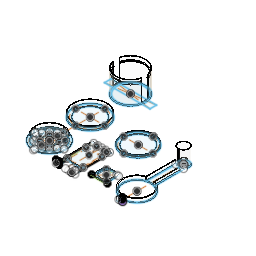
CAPV5 v1 (Autodesk Fusion 360 design; units mm, degrees)
Autodesk Fusion 360 part; units mm, degrees
sketch "Sketch1" plane through (0, 0, 0) normal (0, 0, 1) x (1, 0, 0) in component "Component"
  circle A0 centre (50, 50) radius 41.5
  circle A1 centre (50, 50) radius 18.25
  line L0 (65, 65) -> (35, 65) construction
  line L1 (35, 65) -> (35, 35) construction
  line L2 (35, 35) -> (65, 35) construction
  line L3 (65, 35) -> (65, 65) construction
  line L4 (65, 65) -> (35, 35) construction
  line L5 (35, 65) -> (65, 35) construction
  circle A2 centre (65, 35) radius 1.75
  circle A3 centre (65, 65) radius 1.75
  circle A4 centre (35, 65) radius 1.75
  circle A5 centre (35, 35) radius 1.75
  circle A6 centre (50, 25.5) radius 1.6
  circle A7 centre (50, 74.5) radius 1.6
  line L6 (69.5, 30.5) -> (30.5, 30.5) construction
  line L7 (30.5, 30.5) -> (30.5, 69.5) construction
  line L8 (30.5, 69.5) -> (69.5, 69.5) construction
  line L9 (69.5, 69.5) -> (69.5, 30.5) construction
  line L10 (69.5, 30.5) -> (30.5, 69.5) construction
  line L11 (30.5, 30.5) -> (69.5, 69.5) construction
  line L12 (120, 0) -> (130, 0)
  line L13 (120, 111.4151) -> (120, 0)
  line L14 (169, 0) -> (179, 0)
  line L15 (179, 0) -> (179, 111.4151)
  line L16 (120, 30) -> (179, 30) construction
  line L17 (120, 88) -> (179, 88) construction
  line L18 (125, 0) -> (125, 111.5) construction
  line L19 (174, 0) -> (174, 111.5) construction
  circle A8 centre (125, 30) radius 1.75
  circle A9 centre (174, 30) radius 1.75
  circle A10 centre (125, 88) radius 1.75
  circle A11 centre (174, 88) radius 1.75
  line L20 (50, 50) -> (50, 0) construction
  line L21 (50, 50) -> (50, 93.5) construction
  line L22 (130, 25.5) -> (169, 25.5)
  line L23 (149.5, 111.5) -> (149.5, 0) construction
  line L24 (50, 93.5) -> (50, 225.5598) construction
  circle A12 centre (50, 175.4598) radius 50.1
  circle A13 centre (50, 175.4598) radius 52.1
  circle A14 centre (50, 175.4598) radius 40.1
  circle A15 centre (58.774, 82.7449) radius 5
  circle A16 centre (41.226, 82.7449) radius 5
  circle A17 centre (26.0291, 73.9709) radius 5
  circle A18 centre (17.2551, 58.774) radius 5
  circle A19 centre (17.2551, 41.226) radius 5
  circle A20 centre (26.0291, 26.0291) radius 5
  circle A21 centre (41.226, 17.2551) radius 5
  circle A22 centre (58.774, 17.2551) radius 5
  circle A23 centre (73.9709, 26.0291) radius 5
  circle A24 centre (82.7449, 41.226) radius 5
  circle A25 centre (82.7449, 58.774) radius 5
  circle A26 centre (73.9709, 73.9709) radius 5
  circle A27 centre (65, 35) radius 3
  circle A28 centre (65, 65) radius 3
  circle A29 centre (35, 35) radius 3
  circle A30 centre (35, 65) radius 3
  line L25 (120, 10) -> (130, 10)
  line L26 (169, 10) -> (179, 10)
  line L27 (130, 0) -> (130, 25.5)
  line L28 (169, 25.5) -> (169, 0)
  line L29 (138, 107.4151) -> (138, 111.5) construction
  line L30 (161.05, 107.4151) -> (161.05, 111.5) construction
  line L31 (120, 107.4151) -> (179, 107.4151) construction
  line L32 (120, 111.4151) -> (179, 111.4151)
  circle A31 centre (138, 107.4151) radius 1.7
  circle A32 centre (149.5, 72.4151) radius 1.7
  line L33 (120, 90.4151) -> (179, 90.4151) construction
  circle A33 centre (135.5, 90.4151) radius 1.7
  line L34 (171, 88) -> (171, 30) construction
  line L35 (177, 30) -> (177, 88) construction
  line L36 (122, 30) -> (122, 88) construction
  line L37 (128, 30) -> (128, 88) construction
  line L38 (128, 75.2678) -> (128, 75.2679) construction
  line L39 (128, 75.2678) -> (128, 75.2679)
  circle A34 centre (161.05, 107.4151) radius 1.7
  circle A35 centre (50, 50) radius 50
  circle A36 centre (50, 175.4598) radius 45 construction
  line L40 (50, 175.4598) -> (102.1, 175.4598) construction
  line L41 (50, 175.4598) -> (-2.1, 175.4598) construction
  circle A37 centre (50, 220.4598) radius 1.6
  circle A38 centre (95, 175.4598) radius 1.6
  circle A39 centre (50, 130.4598) radius 1.6
  circle A40 centre (5, 175.4598) radius 1.6
  circle A41 centre (50, 50) radius 45 construction
  circle A42 centre (50, 95) radius 2.05
  circle A43 centre (4.9633, 50.0341) radius 2.05
  circle A44 centre (49.9642, 4.9627) radius 2.05
  circle A45 centre (95.0328, 50.0188) radius 2.05
  arc A46 (48.6263, 93.4783) -> (6.5215, 51.3662) centre (50, 50) ccw
  arc A47 (6.5193, 48.6993) -> (48.6327, 6.5214) centre (50, 50) ccw
  arc A48 (51.2973, 6.52) -> (93.4763, 48.6847) centre (50.0149, 49.9818) ccw
  arc A49 (93.4741, 51.3504) -> (51.333, 93.4426) centre (50.0149, 49.9818) ccw
  circle A50 centre (50, 50) radius 33.9 construction
  circle A51 centre (50, 50) radius 38.9 construction
  circle A52 centre (198.4118, 175.4598) radius 45 construction
  line L42 (198.4118, 175.4598) -> (247.9118, 175.4598) construction
  circle A53 centre (198.4118, 175.4598) radius 40.1
  circle A54 centre (243.4118, 175.4598) radius 1.6
  circle A55 centre (198.4118, 130.4598) radius 1.6
  circle A56 centre (198.4118, 220.4598) radius 1.6
  circle A57 centre (153.4118, 175.4598) radius 1.6
  circle A58 centre (198.4118, 175.4598) radius 49.5
  line L43 (198.4118, 175.4598) -> (148.9118, 175.4598) construction
  circle A59 centre (198.4118, 175.4598) radius 47.6
  circle A60 centre (168.5, 107.4151) radius 1.7
  line L44 (320, 50) -> (320, -0.2775) construction
  line L45 (321.5, 8.5271) -> (321.5, -6.2719)
  line L46 (318.5, 8.5271) -> (318.5, -6.2719)
  arc A61 (321.5, 8.5271) -> (318.5, 8.5271) centre (320, 50) ccw
  line L47 (314.5, 5.8412) -> (314.5, -6.2719)
  line L48 (325.5, 5.8412) -> (325.5, -6.2719)
  line L49 (314.5, -6.2719) -> (318.5, -6.2719)
  line L50 (321.5, -6.2719) -> (325.5, -6.2719)
  line L51 (314, -0.2719) -> (327, -0.2719) construction
  line L52 (320, 50) -> (320, 193.7281) construction
  line L53 (317, 193.7281) -> (323, 193.7281)
  circle A62 centre (320.0004, 193.6763) radius 7.45
  line L54 (332, 89.7272) -> (332, 181.6865)
  line L55 (308, 89.7272) -> (308, 181.6865)
  arc A63 (322, 178.862) -> (318, 178.862) centre (320, 193.7281) ccw
  arc A64 (322, 176.8462) -> (318, 176.8462) centre (320, 193.7281) ccw
  line L56 (334, 92.2404) -> (334, 184.0845)
  line L57 (306, 92.2404) -> (306, 184.0845)
  arc A65 (325.5, 5.8412) -> (334, 92.2404) centre (320, 50) ccw
  arc A66 (306, 92.2404) -> (314.5, 5.8412) centre (320, 50) ccw
  arc A67 (332, 92.8515) -> (308, 92.8515) centre (320, 50) ccw
  circle A68 centre (320, 193.7281) radius 9.5
  line L58 (318, 176.8462) -> (322, 176.8462)
  line L59 (318, 178.862) -> (322, 178.862)
  line L60 (322, 176.8462) -> (322, 178.862)
  line L61 (322, 184.441) -> (322, 186.4997)
  line L62 (318, 176.8462) -> (318, 178.862)
  line L63 (318, 184.441) -> (318, 186.4999)
  line L64 (251, 28.5) -> (257.5, 28.5)
  line L65 (229.5, 65) -> (229.5, 21.5) construction
  line L66 (245.5, 62) -> (245.5, 30) construction
  circle A69 centre (245.5, 30) radius 2.75
  line L67 (213.5, 62) -> (213.5, 30) construction
  circle A70 centre (213.5, 62) radius 2.75
  line L68 (208, 28.5) -> (208, 66.5)
  line L69 (213.5, 30) -> (245.5, 62) construction
  line L70 (208, 62) -> (251, 62) construction
  line L71 (245.5, 30) -> (213.5, 62) construction
  line L72 (251, 28.5) -> (251, 66.5)
  circle A71 centre (125, 30) radius 3
  circle A72 centre (174, 30) radius 3
  circle A73 centre (125, 88) radius 3
  circle A74 centre (174, 88) radius 3
  line L73 (208, 30) -> (251, 30) construction
  line L74 (208, 66.5) -> (251, 66.5)
  circle A75 centre (229.5, 46) radius 19
  circle A76 centre (50, 300) radius 44.25
  circle A77 centre (50, 300) radius 46.25
  circle A78 centre (50, 300) radius 41.25
  line L75 (120, 290) -> (-20, 290)
  line L76 (-20, 290) -> (-20, 310)
  line L77 (-20, 310) -> (120, 310)
  line L78 (120, 310) -> (120, 290)
  line L79 (120, 290) -> (-20, 310) construction
  line L80 (-20, 290) -> (120, 310) construction
  line L81 (201.5, 25) -> (257.5, 25) construction
  circle A79 centre (205, 25) radius 1.4
  circle A80 centre (254, 25) radius 1.4
  line L82 (201.5, 21.5) -> (257.5, 21.5)
  line L83 (257.5, 28.5) -> (257.5, 21.5)
  line L84 (251, 28.5) -> (201.5, 28.5) construction
  line L85 (208, 28.5) -> (201.5, 28.5)
  line L86 (201.5, 28.5) -> (201.5, 21.5)
  arc A81 (53.6265, 93.3123) -> (46.3574, 93.3472) centre (50, 95) ccw
  arc A82 (6.6542, 53.6591) -> (6.6486, 46.4064) centre (4.9633, 50.0341) ccw
  arc A83 (46.3394, 6.6542) -> (53.5916, 6.6484) centre (49.9642, 4.9627) ccw
  arc A84 (93.3472, 46.3913) -> (93.3412, 53.6436) centre (95.0328, 50.0188) ccw
  point P0 (50, 50)
  point P1 (50, 50)
  point P2 (50, 25.5)
  point P3 (50, 74.5)
  point P4 (50, 25.5)
  point P5 (50, 74.5)
  point P6 (50, 50)
  point P7 (120, 0)
  point P8 (169, 0)
  point P9 (149.5, 72.4151)
  point P10 (50, 50)
  point P11 (198.4118, 223.0598)
  point P12 (168.5, 107.4151)
  point P13 (320, 50)
  point P14 (320, 50)
  point P15 (50, 300)
  dimension "d3" = 83
  dimension "d4" = 36.5
  dimension "d12" = 30
  dimension "d13" = 30
  dimension "d14" = 3.5
  dimension "d15" = 3.5
  dimension "d16" = 3.5
  dimension "d17" = 3.5
  dimension "d18" = 24.5
  dimension "d19" = 24.5
  dimension "d28" = 3.2
  dimension "d29" = 3.2
  dimension "d30" = 39
  dimension "d31" = 39
  dimension "d61" = 10
  dimension "d63" = 10
  dimension "d66" = 30
  dimension "d67" = 58
  dimension "d68" = 3.5
  dimension "d69" = 3.5
  dimension "d70" = 3.5
  dimension "d71" = 3.5
  dimension "d80" = 49
  dimension "d93" = 4.5
  dimension "d109" = 87
  dimension "d110" = 100.2
  dimension "d111" = 104.2
  dimension "d112" = 80.2
  dimension "d120" = 77.8
  dimension "d123" = 6
  dimension "d124" = 6
  dimension "d125" = 6
  dimension "d126" = 6
  dimension "d150" = 4
  dimension "d151" = 3.4
  dimension "d153" = 35
  dimension "d154" = 3.4
  dimension "d166" = 3.4
  dimension "d190" = 3.4
  dimension "d199" = 100
  dimension "d200" = 90
  dimension "d201" = 3.2
  dimension "d202" = 3.2
  dimension "d203" = 3.2
  dimension "d204" = 3.2
  dimension "d205" = 90
  dimension "d206" = 4.1
  dimension "d222" = 95.2
  dimension "d223" = 99
  dimension "d224" = 80.2
  dimension "d225" = 90
  dimension "d226" = 3.2
  dimension "d227" = 3.2
  dimension "d228" = 3.2
  dimension "d229" = 3.2
  dimension "d243" = 33
  dimension "d244" = 3.4
  dimension "d248" = 10.5
  dimension "d249" = 17
  dimension "d250" = 83
  dimension "d251" = 89
  dimension "d254" = 4
  dimension "d255" = 4
  dimension "d260" = 200
  dimension "d261" = 30
  dimension "d265" = 14.9
  dimension "d266" = 19
  dimension "d267" = 2
  dimension "d268" = 2
  dimension "d270" = 34
  dimension "d316" = 10
  dimension "d353" = 16
  dimension "d354" = 5.5
  dimension "d357" = 5.5
  dimension "d358" = 38
  dimension "d371" = 6
  dimension "d372" = 6
  dimension "d373" = 6
  dimension "d374" = 6
  dimension "d389" = 88.5
  dimension "d390" = 92.5
  dimension "d391" = 82.5
  dimension "d409" = 20
  dimension "d416" = 2.8
  dimension "d418" = 2.8
  dimension "d421" = 3.5
  dimension "d423" = 3.5
  dimension "d424" = 3.5
  dimension "d425" = 3.5
  dimension "d432" = 24.5
  dimension "d433" = 24.5
  dimension "d434" = 45
  dimension "d435" = 4.1
  dimension "d436" = 4.1
  dimension "d437" = 4.1
  dimension "d442" = 8
  dimension "d443" = 8
  dimension "d444" = 8
  dimension "d445" = 8
  constraint coincident P10 P6
  constraint concentric A0 A1
  constraint horizontal L0
  constraint perpendicular L0 L1
  constraint parallel L0 L2
  constraint parallel L1 L3
  constraint coincident L4 P10
  constraint coincident L5 P10
  constraint coincident L2.end L3.start
  constraint coincident L0.start L3.end
  constraint coincident L0.end L1.start
  constraint coincident L1.end L2.start
  constraint coincident P4 P2
  constraint coincident P5 P3
  constraint horizontal L6
  constraint perpendicular L6 L7
  constraint parallel L6 L8
  constraint parallel L7 L9
  constraint coincident L10 P10
  constraint coincident L11 P10
  constraint horizontal P7 P8
  constraint horizontal L12
  constraint vertical L27
  constraint vertical L13
  constraint coincident P7 L12.start
  constraint horizontal L14
  constraint vertical L15
  constraint coincident P8 L14.start
  constraint coincident L13 L16.start
  constraint coincident L15 L16.end
  constraint perpendicular L15 L16
  constraint coincident L13 L17.start
  constraint coincident L15 L17.end
  constraint perpendicular L15 L17
  constraint midpoint L12 L18.start
  constraint midpoint L14 L19.start
  constraint coincident L18 A8.centre
  constraint coincident L16 A8.centre
  constraint coincident L19 A9.centre
  constraint coincident L16 A9.centre
  constraint coincident L17 A10.centre
  constraint coincident L18 A10.centre
  constraint coincident L17 A11.centre
  constraint coincident L19 A11.centre
  constraint perpendicular L2 L20
  constraint vertical L21
  constraint perpendicular L16 L23
  constraint parallel L21 L24
  constraint coincident L24 A12.centre
  constraint concentric A12 A13
  constraint concentric A13 A14
  constraint concentric A1 A51
  constraint concentric A2 A27
  constraint concentric A3 A28
  constraint concentric A5 A29
  constraint concentric A4 A30
  constraint coincident L13 L25.start
  constraint coincident L15 L26.end
  constraint perpendicular L15 L25
  constraint coincident L25.end L27
  constraint collinear L25 L26
  constraint coincident L13 L31.start
  constraint coincident L15 L31.end
  constraint perpendicular L15 L31
  constraint perpendicular L15 L32
  constraint coincident L31 L29.start
  constraint coincident L23 P9
  constraint coincident P9 A32.centre
  constraint coincident L13 L33.start
  constraint coincident L15 L33.end
  constraint perpendicular L15 L33
  constraint coincident L17 L34.start
  constraint coincident L16 L34.end
  constraint coincident L16 L35.start
  constraint coincident L17 L35.end
  constraint coincident L16 L36.start
  constraint coincident L17 L36.end
  constraint coincident L16 L37.start
  constraint coincident L37 L38.start
  constraint coincident L37 L38.end
  constraint coincident L31 L30.start
  constraint concentric A12 A36
  constraint coincident A12 L24.end
  constraint coincident A12.centre A13.centre
  constraint coincident A13 L40.end
  constraint horizontal L40
  constraint coincident A13 L41.end
  constraint horizontal L41
  constraint coincident A36 A37.centre
  constraint coincident L24 A37.centre
  constraint coincident A36 A38.centre
  constraint coincident L40 A38.centre
  constraint coincident A36 A39.centre
  constraint coincident L24 A39.centre
  constraint coincident A36 A40.centre
  constraint coincident L41 A40.centre
  constraint concentric A0 A41
  constraint coincident A41 A42.centre
  constraint coincident L24 A42.centre
  constraint concentric A46 A47
  constraint concentric A48 A49
  constraint coincident A45 A48.end
  constraint coincident A45 A49.start
  constraint coincident A44 A48.start
  constraint coincident A44 A47.end
  constraint coincident A43 A47.start
  constraint coincident A43 A46.end
  constraint coincident A42 A49.end
  constraint coincident A42 A46.start
  constraint coincident A26.centre A50
  constraint concentric A58 A59
  constraint concentric A53 A58
  constraint concentric A52 A59
  constraint coincident P11 A59
  constraint coincident A52.centre L42.start
  constraint coincident L42.end A58
  constraint horizontal L42
  constraint coincident L43.end A58
  constraint horizontal L43
  constraint coincident A56.centre A52
  constraint coincident A54.centre A52
  constraint coincident A54.centre L42
  constraint coincident A55.centre A52
  constraint coincident A57.centre A52
  constraint coincident A57.centre L43
  constraint coincident L31 P12
  constraint coincident P12 A60.centre
  constraint concentric A61 A65
  constraint coincident P14 P13
  constraint vertical L44
  constraint vertical L45
  constraint vertical L46
  constraint perpendicular L48 L49
  constraint coincident L45.end L49
  constraint collinear L49 L50
  constraint perpendicular L44 L51
  constraint parallel L44 L52
  constraint coincident L52.end A63.centre
  constraint perpendicular L53 L60
  constraint coincident A67.end A65
  constraint coincident A67.start A65
  constraint concentric A63 A64
  constraint coincident A64 L56.end
  constraint coincident A64 L57.end
  constraint coincident L57.start A65
  constraint concentric A65 A67
  constraint concentric A66 A67
  constraint coincident A62 L61.end
  constraint coincident A62 L63.end
  constraint coincident A68 L61.start
  constraint collinear L60 L61
  constraint coincident A68 L63.start
  constraint collinear L62 L63
  constraint coincident A61 L55.start
  constraint coincident L55 A67.end
  constraint coincident A61 L54.start
  constraint coincident L54 A67.start
  constraint coincident L67.start L70
  constraint coincident L66.start L70
  constraint perpendicular L66 L70
  constraint coincident L67.start A70.centre
  constraint coincident L66.end A69.centre
  constraint perpendicular L69 L71
  constraint midpoint A75.centre L69
  constraint concentric A8 A71
  constraint concentric A9 A72
  constraint concentric A10 A73
  constraint concentric A11 A74
  constraint coincident L68 L70.start
  constraint coincident L68 L73.start
  constraint concentric A76 A77
  constraint concentric A76 A78
  constraint horizontal L75
  constraint perpendicular L75 L76
  constraint parallel L75 L77
  constraint parallel L76 L78
  constraint coincident L79 P15
  constraint coincident L80 P15
  constraint coincident P15 A76.centre
  constraint perpendicular L67 L81
  constraint coincident L81 A79.centre
  constraint coincident L81 A80.centre
  constraint horizontal L82
  constraint perpendicular L82 L83
  constraint coincident L83 L81.end
  constraint perpendicular L68 L84
  constraint coincident L84 L68.start
  constraint perpendicular L82 L86
  constraint coincident L86 L81.start
  constraint coincident L82 L65.end
  constraint coincident L72 L73.end
  constraint coincident A75 L65.start
  constraint coincident A46 A81.end
  constraint coincident A49 A81.start
  constraint concentric A43 A82
  constraint coincident A46 A82.start
  constraint coincident A47 A82.end
  constraint concentric A44 A83
  constraint coincident A47 A83.start
  constraint coincident A48 A83.end
  constraint concentric A45 A84
  constraint coincident A49 A84.end
  constraint coincident A48 A84.start
  measures "d3" diameter of A0
  measures "d4" diameter of A1
  measures "d12" distance of L1.end L2.end
  measures "d13" distance of L0.end L1.end
  measures "d14" diameter of A2
  measures "d15" diameter of A3
  measures "d16" diameter of A4
  measures "d17" diameter of A5
  measures "d18" distance of P10 P4
  measures "d19" distance of P10 P5
  measures "d28" diameter of A6
  measures "d29" diameter of A7
  measures "d30" distance of L7.end L8.end
  measures "d31" distance of L6.end L7.end
  measures "d61" distance of P7 L12.end
  measures "d63" distance of P8 L14.end
  measures "d66" distance of L14.end L16.end
  measures "d67" distance of L16.end L17.end
  measures "d68" diameter of A8
  measures "d69" diameter of A9
  measures "d70" diameter of A10
  measures "d71" diameter of A11
  measures "d80" distance of L18.start L19.start
  measures "d93" distance of L16 L22
  measures "d109" diameter of A46
  measures "d110" diameter of A12
  measures "d111" diameter of A13
  measures "d112" diameter of A14
  measures "d120" diameter of A51
  measures "d123" diameter of A27
  measures "d124" diameter of A28
  measures "d125" diameter of A29
  measures "d126" diameter of A30
  measures "d150" distance of L15.end L31.end
  measures "d151" diameter of A31
  measures "d153" distance of L31 P9
  measures "d154" diameter of A32
  measures "d166" diameter of A33
  measures "d190" diameter of A34
  measures "d199" diameter of A35
  measures "d200" diameter of A36
  measures "d201" diameter of A37
  measures "d202" diameter of A38
  measures "d203" diameter of A39
  measures "d204" diameter of A40
  measures "d205" diameter of A41
  measures "d206" diameter of A42
  measures "d222" diameter of A59
  measures "d223" diameter of A58
  measures "d224" diameter of A53
  measures "d225" diameter of A52
  measures "d226" diameter of A56
  measures "d227" diameter of A54
  measures "d228" diameter of A55
  measures "d229" diameter of A57
  measures "d243" horizontal distance of A33.centre P12
  measures "d244" diameter of A60
  measures "d248" distance of L18 A33.centre
  measures "d249" distance of L31 L33
  measures "d250" diameter of A61
  measures "d251" diameter of A65
  measures "d254" distance of L46 L47
  measures "d255" distance of L45 L48
  measures "d260" vertical distance of L48.end L52.end
  measures "d261" diameter of A63
  measures "d265" diameter of A62
  measures "d266" diameter of A68
  measures "d267" distance of L52 L60
  measures "d268" distance of L52 L62
  measures "d270" diameter of A64
  measures "d316" distance of L54 L60
  measures "d353" distance of L65 L67
  measures "d354" diameter of A70
  measures "d357" diameter of A69
  measures "d358" diameter of A75
  measures "d371" diameter of A71
  measures "d372" diameter of A72
  measures "d373" diameter of A73
  measures "d374" diameter of A74
  measures "d389" diameter of A76
  measures "d390" diameter of A77
  measures "d391" diameter of A78
  measures "d409" distance of L75.end L76.end
  measures "d416" diameter of A79
  measures "d418" diameter of A80
  measures "d421" distance of L81 L82
  measures "d423" distance of A80.centre L83
  measures "d424" distance of L64 A80.centre
  measures "d425" distance of A79.centre L86
  measures "d432" horizontal distance of A79.centre L65.end
  measures "d433" horizontal distance of A80.centre L65.end
  measures "d434" vertical distance of L72.end L82.end
  measures "d435" diameter of A45
  measures "d436" diameter of A43
  measures "d437" diameter of A44
  measures "d442" diameter of A81
  measures "d443" diameter of A82
  measures "d444" diameter of A83
  measures "d445" diameter of A84
extrude "Extrude7" add sketch "Sketch1" along normal blind 2 contours A0 makes body 1 in component "Component"
extrude "Extrude35" add sketch "Sketch1" along normal blind 13.5 contours A1 A28 | A1 A28 | A1 A27 | A1 A27 | A1 A30 | A1 A30 | A1 A29 | A1 A29 | A2 | A3 | A4 | A5 bodies 1 in component "Component"
extrude "Extrude36" cut sketch "Sketch1" along normal blind 6.5 from surface at 7 contours A2 | A3 | A4 | A5 bodies 1 in component "Component"
extrude "Extrude13" add sketch "Sketch1" along normal blind 18 contours A42 A43 A44 A45 A46 A47 A48 A49 bodies 1 in component "Component"
extrude "Extrude39" add sketch "Sketch1" along normal blind 6 contours A42 A46 A49 A81 | A43 A46 A47 A82 | A45 A48 A49 A84 | A44 A47 A48 A83 bodies 1 in component "Component"
extrude "Extrude37" add sketch "Sketch1" along normal blind 2 contours A0 | A1 A28 | A1 A27 | A1 A30 | A1 A29 | A2 | A3 | A4 | A5 | A35 | A42 A46 A49 A81 | A42 A43 A44 A45 A46 A47 A48 A49 | A43 A46 A47 A82 | A45 A48 A49 A84 | A44 A47 A48 A83 picked at (63.6381, 62.8117) picked at (63.6381, 37.1883) picked at (36.3608, 62.8111) picked at (36.3608, 37.1889) bodies 1 in component "Component"
extrude "Extrude12" add sketch "Sketch1" along normal blind 10 separate body contours L12 L13 L25 L27 | L14 L15 L26 L28 makes body 2 at (120, 6.6667, 3.3333) makes body 3 at (179, 3.3333, 3.3333) in component "Component"
extrude "Extrude18" add sketch "Sketch1" along normal blind 3 contours L13 L15 L22 L25 L26 L27 L28 L32 bodies 2 3 in component "Component"
extrude "Extrude5" add sketch "Sketch1" along normal blind 3 contours L13 L15 L22 L25 L26 L27 L28 L32 | A71 | A72 | A73 | A74 bodies 2 in component "Component"
extrude "Extrude14" add sketch "Sketch1" along normal blind 6 contours A71 | A72 | A73 | A74 bodies 2 in component "Component"
sketch "Sketch3" plane through (0, 0, 0) normal (0, -1, 0) x (1, 0, 0) in component "Component"
  line L0 (120, 0) -> (130, 0)
  line L1 (130, 0) -> (130, 10)
  line L2 (130, 10) -> (120, 10)
  line L3 (120, 10) -> (120, 0)
  line L4 (120, 0) -> (130, 10) construction
  line L5 (130, 0) -> (120, 10) construction
  line L6 (159, 0) -> (169, 0) construction
  line L7 (169, 0) -> (169.0001, 0.0001) construction
  circle A0 centre (125, 5) radius 2.05
  line L8 (169, 0) -> (179, 10) construction
  line L9 (179, 0) -> (169, 10) construction
  circle A1 centre (174, 5) radius 2.05
  point P0 (169, 0)
  dimension "d89" = 4.1
  dimension "d333" = 4.1
  constraint coincident L0.start L3.end
  constraint coincident L1.end L2.start
  constraint coincident L0.end L1.start
  constraint coincident L2.end L3.start
  constraint coincident P0 L6.end
  constraint midpoint L4 A0.centre
  constraint midpoint L9 A1.centre
  measures "d89" diameter of A0
  measures "d333" diameter of A1
extrude "Extrude16" cut sketch "Sketch3" against normal blind 12 contours A0 bodies 2 in component "Component"
extrude "Extrude1" cut sketch "Sketch3" against normal blind 12 contours A1 bodies 2 in component "Component"
extrude "Extrude21" add sketch "Sketch1" along normal blind 12 separate body contours A13 makes body 4 in component "Component"
extrude "Extrude22" add sketch "Sketch1" along normal blind 2 contours A12 | A37 | A38 | A39 | A40 bodies 4 in component "Component"
extrude "Extrude40" cut sketch "Sketch1" along normal blind 2 contours A37 | A38 | A39 | A40 bodies 4 in component "Component"
extrude "Extrude41" add sketch "Sketch1" along normal blind 2 separate body contours A59 makes body 5 in component "Component"
extrude "Extrude42" add sketch "Sketch1" along normal blind 4 contours A58 bodies 5 in component "Component"
extrude "Extrude7'" add sketch "Sketch1" along normal blind 2 separate body contours A78 L77 | A78 L75 L77 | A78 L75 makes body 6 in component "Component"
extrude "Extrude8" add sketch "Sketch1" along normal blind 2 contours A76 A78 L75 L77 | A76 A78 L77 | A76 A78 L75 | A76 A78 L75 L77 bodies 6 in component "Component"
extrude "Extrude9" add sketch "Sketch1" along normal blind 70 contours A76 A77 L75 L77 | A76 A77 L77 | A76 A77 L75 | A76 A77 L75 L77 bodies 6 in component "Component"
extrude "Extrude10" add sketch "Sketch1" along normal blind 5 from surface at 55 contours A76 A78 L75 L77 | A76 A78 L77 | A76 A78 L75 | A76 A78 L75 L77 bodies 6 in component "Component"
chamfer "Chamfer2" distance 3 angle 45 1 edges at (11.5415, 314.9166, 55) on bodies 6 in component "Component"
extrude "Extrude11" cut sketch "Sketch1" along normal blind 65 from surface at 5 contours A76 A78 L75 L77 | A76 A77 L75 L77 | A76 A78 L75 L77 | A76 A77 L75 L77 bodies 6 in component "Component"
extrude "Extrude68" add sketch "Sketch1" along normal blind 3 separate body contours L64 L68 L72 L74 L82 L83 L85 L86 makes body 7
copy_body "CutPasteBodies1" bodies 7 removing the originals makes body 8 in component "Component"
extrude "Extrude15" add sketch "Sketch1" along normal blind 3 separate body contours A61 L54 L55 A67 | L54 L55 A64 A67 L58 | L58 L59 L60 L62 | A63 L59 | A62 | A62 A68 L61 L63 picked at (320, 184.91) makes body 9 in component "Component"
extrude "Extrude16'" add sketch "Sketch1" along normal blind 12 contours L45 A61 L48 L50 L54 A64 L56 A65 | L46 A61 L47 L49 L55 A64 L57 A66 | A62 A68 L61 L63 picked at (314.5297, 200.6029) bodies 9 in component "Component"
extrude "Extrude17" add sketch "Sketch1" along normal blind 50 contours A63 A64 L60 L62 bodies 9 in component "Component"
sketch "Sketch4" plane through (325.5, 0, 0) normal (1, 0, 0) x (0, 1, 0) in component "Component"
  line L0 (-6.2719, 0) -> (5.8412, 0)
  line L1 (5.8412, 0) -> (5.8412, 12)
  line L2 (5.8412, 12) -> (-6.2719, 12)
  line L3 (-6.2719, 12) -> (-6.2719, 0)
  line L4 (0, 0) -> (0, 12) construction
  line L5 (-6.2719, 6) -> (5.8412, 6) construction
  circle A0 centre (-0.2153, 6) radius 1.75
  dimension "d462" = 3.5
  constraint coincident L4.start origin
  constraint coincident L2 L4.end
  constraint perpendicular L2 L4
  constraint midpoint L3 L5.start
  constraint midpoint L1 L5.end
  constraint midpoint L5 A0.centre
  measures "d462" diameter of A0
extrude "Extrude18'" cut sketch "Sketch4" against normal blind 15 contours A0 bodies 9 in component "Component"
extrude "Extrude14'" [suppressed] in component "Component"
component "Component" placed x (1, 0, 0) y (0, 1, 0) z (0, 0, 1) at (0, 0, 0)
equation "d18 = ( 49 / 2 ) * 1 mm"
equation "d19 = ( 49 / 2 ) * 1 mm"
equation "d432 = ( 49 / 2 ) * 1 mm"
equation "d433 = ( 49 / 2 ) * 1 mm"
named bodies: "cap-main", "cap-support", "cap-right-support", "cap-dome-holder", "cap-gasket-template", "cap-base-holder", "cap-fan-holder", "cap-weather-shield"
